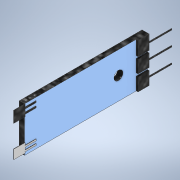
# Autodesk Inventor part: SENSOR
Saved by Autodesk Inventor 2021 (Build 250183000, 183)
## iProperties
Created: 2021-07-10
Part Number: SENSOR
Material: Generic
Document SubType Name: Modeling
Designer: HP
Density: 1 g/cm^3
Appearance: Black Cast
Author: HP
Autodesk Inventor part; units mm, degrees
ref_plane "YZ Plane" through (0, 0, 0) normal (1, 0, 0) x (0, 1, 0)
ref_plane "XZ Plane" through (0, 0, 0) normal (0, 1, 0) x (-1, 0, 0)
ref_plane "XY Plane" through (0, 0, 0) normal (0, 0, 1) x (1, 0, 0)
sketch "Sketch1" plane through (0, 0, 0) normal (1, 0, 0) x (0, 1, 0)
  line L0 (3.175, 7.9375) -> (-3.175, 7.9375)
  line L1 (-3.175, 7.9375) -> (-3.175, -9.525)
  line L2 (-3.175, -9.525) -> (3.175, -9.525)
  line L3 (3.175, -9.525) -> (3.175, 7.9375)
  line L4 (3.175, -8.3415) -> (1.4145, -8.3415)
  line L5 (1.4145, -8.3415) -> (1.4145, -9.525)
  line L6 (1.4145, -9.525) -> (3.175, -9.525)
  line L7 (3.175, -9.525) -> (3.175, -8.3415)
  line L8 (1.113, -8.3415) -> (-0.7652, -8.3415)
  line L9 (-0.7652, -8.3415) -> (-0.7652, -9.525)
  line L10 (-0.7652, -9.525) -> (1.113, -9.525)
  line L11 (1.113, -9.525) -> (1.113, -8.3415)
  line L12 (-1.2985, -8.3415) -> (-3.175, -8.3415)
  line L13 (-3.175, -8.3415) -> (-3.175, -9.525)
  line L14 (-3.175, -9.525) -> (-1.2985, -9.525)
  line L15 (-1.2985, -9.525) -> (-1.2985, -8.3415)
  point P0 (0, 0)
  constraints: 32 end point, 8 parallel, 4 horizontal, 4 perpendicular, 3 point on line
extrude "Extrusion1" add sketch "Sketch1" along normal blind 0.762
sketch "Sketch2" plane through (0.762, 0, 0) normal (1, 0, 0) x (0, 0, -1)
  line L0 (9.525, 3.175) -> (-7.9375, 3.175) projected
  line L1 (9.525, -3.175) -> (9.525, 3.175) projected
  line L2 (7.9375, 3.175) -> (9.525, 3.175)
  line L3 (9.525, 3.175) -> (9.525, 1.1594)
  line L4 (9.525, 1.1594) -> (7.9375, 1.1594)
  line L5 (7.9375, 1.1594) -> (7.9375, 3.175)
  line L6 (7.9375, 0.8348) -> (9.525, 0.8348)
  line L7 (9.525, 0.8348) -> (9.525, -0.9507)
  line L8 (9.525, -0.9507) -> (7.9375, -0.9507)
  line L9 (7.9375, -0.9507) -> (7.9375, 0.8348)
  line L10 (7.9375, -1.3449) -> (9.525, -1.3449)
  line L11 (9.525, -1.3449) -> (9.525, -3.175)
  line L12 (9.525, -3.175) -> (7.9375, -3.175)
  line L13 (7.9375, -3.175) -> (7.9375, -1.3449)
  point P0 (0, 0)
  constraints: 24 end point, 6 parallel, 3 horizontal, 3 perpendicular, 3 point on line
extrude "Extrusion2" add sketch "Sketch2" along normal blind 0.254
sketch "Sketch3" plane through (1.016, 0, 0) normal (1, 0, 0) x (0, 0, -1)
  line L0 (9.525, 2.2739) -> (12.7, 2.2739)
  line L1 (12.7, 2.2739) -> (12.7, 2.0961)
  line L2 (12.7, 2.0961) -> (9.525, 2.0961)
  line L3 (9.525, 2.0961) -> (9.525, 2.2739)
  line L4 (9.525, -3.175) -> (9.525, 3.175) projected
  line L5 (9.525, 0) -> (12.7, 0)
  line L6 (12.7, 0) -> (12.7, 0.1856)
  line L7 (12.7, 0.1856) -> (9.525, 0.1856)
  line L8 (9.525, 0.1856) -> (9.525, 0)
  line L9 (9.525, -1.9723) -> (12.7, -1.9723)
  line L10 (12.7, -1.9723) -> (12.7, -2.1501)
  line L11 (12.7, -2.1501) -> (9.525, -2.1501)
  line L12 (9.525, -2.1501) -> (9.525, -1.9723)
  point P0 (0, 0)
  dimension "d4" = 0.1778
  dimension "d5" = 0.1778
  constraints: 24 end point, 6 parallel, 3 horizontal, 3 perpendicular, 1 midpoint, 1 point on line
  measures "d4" distance of L0.end L1.end
  measures "d5" distance of L9.end L10.end
extrude "Extrusion3" add sketch "Sketch3" along normal blind 0.0508
sketch "Sketch4" plane through (0.762, 0, 0) normal (1, 0, 0) x (0, 0, -1)
  circle A0 centre (5.4047, 0) radius 0.6422
  point P0 (0, 0)
  constraints: 1 centre point
extrude "Extrusion4" cut sketch "Sketch4" against normal mid plane 25.4
sketch "Sketch5" plane through (0.762, 0, 0) normal (1, 0, 0) x (0, 0, -1)
  line L0 (-7.9375, 3.175) -> (-7.9375, -3.175) projected
  line L1 (-7.9375, 2.7765) -> (-6.35, 2.7765)
  line L2 (-6.35, 2.7765) -> (-6.35, 2.5479)
  line L3 (-6.35, 2.5479) -> (-7.9375, 2.5479)
  line L4 (-7.9375, 2.5479) -> (-7.9375, 2.7765)
  line L5 (-7.9375, 2.1295) -> (-6.35, 2.1295)
  line L6 (-6.35, 2.1295) -> (-6.35, 1.9009)
  line L7 (-6.35, 1.9009) -> (-7.9375, 1.9009)
  line L8 (-7.9375, 1.9009) -> (-7.9375, 2.1295)
  line L9 (-7.9375, -2.7226) -> (-6.35, -2.7226)
  line L10 (-6.35, -2.7226) -> (-6.35, -2.494)
  line L11 (-6.35, -2.494) -> (-7.9375, -2.494)
  line L12 (-7.9375, -2.494) -> (-7.9375, -2.7226)
  line L13 (-7.9375, -2.1565) -> (-6.35, -2.1565)
  line L14 (-6.35, -2.1565) -> (-6.35, -1.9279)
  line L15 (-6.35, -1.9279) -> (-7.9375, -1.9279)
  line L16 (-7.9375, -1.9279) -> (-7.9375, -2.1565)
  point P0 (0, 0)
  dimension "d10" = 0.2286
  dimension "d11" = 0.2286
  dimension "d12" = 0.2286
  dimension "d13" = 0.2286
  constraints: 32 end point, 8 parallel, 4 horizontal, 4 perpendicular, 4 point on line
  measures "d10" distance of L1.end L2.end
  measures "d11" distance of L5.end L6.end
  measures "d12" distance of L10.end L9.end
  measures "d13" distance of L14.end L13.end
extrude "Extrusion5" add sketch "Sketch5" along normal blind 0.0508
sketch "Sketch6" plane through (0.762, 0, 0) normal (1, 0, 0) x (0, 0, -1)
  line L0 (-7.9375, 3.175) -> (-7.9375, -3.175) projected
  line L1 (-7.9375, 1.5875) -> (-9.525, 1.5875)
  line L2 (-9.525, 1.5875) -> (-9.525, 3.175)
  line L3 (-9.525, 3.175) -> (-7.9375, 3.175)
  line L4 (-7.9375, 3.175) -> (-7.9375, 1.5875)
  line L5 (-7.9375, -2.8843) -> (-9.525, -2.8843)
  line L6 (-9.525, -2.8843) -> (-9.525, -1.5875)
  line L7 (-9.525, -1.5875) -> (-7.9375, -1.5875)
  line L8 (-7.9375, -1.5875) -> (-7.9375, -2.8843)
  point P0 (0, 0)
  constraints: 16 end point, 4 parallel, 2 horizontal, 2 perpendicular, 2 point on line
extrude "Extrusion6" add sketch "Sketch6" along normal blind 0.0508
body "Solid1"
